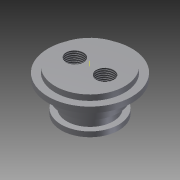
# Autodesk Inventor part: GL45 bottle cap insert with npt fittings
Saved by Autodesk Inventor 2011 (Build 150239000, 239)
## iProperties
Created: 2012-03-14
Part Number: GL45 bottle cap insert with npt fittings
Document SubType Name: Modeling
Designer: Marc
Density: 1 g/cm^3
Author: Marc
Autodesk Inventor part; units mm, degrees
ref_plane "YZ Plane" through (0, 0, 0) normal (1, 0, 0) x (0, 1, 0)
ref_plane "XZ Plane" through (0, 0, 0) normal (0, 1, 0) x (-1, 0, 0)
ref_plane "XY Plane" through (0, 0, 0) normal (0, 0, 1) x (1, 0, 0)
sketch "Sketch1" plane through (0, 0, 0) normal (0, 0, 1) x (1, 0, 0)
  line L0 (0, 0) -> (-14.478, 0)
  line L1 (-14.478, 0) -> (-14.478, 2.54)
  line L2 (-14.478, 2.54) -> (-11.684, 2.54)
  line L3 (-11.684, 2.54) -> (-11.684, 7.62)
  line L4 (-11.684, 7.62) -> (-14.478, 7.62)
  line L5 (-14.478, 7.62) -> (-14.478, 15.24)
  line L6 (-14.478, 15.24) -> (-21.082, 15.24)
  line L7 (-21.082, 15.24) -> (-21.082, 18.034)
  line L8 (-21.082, 18.034) -> (-17.526, 18.034)
  line L9 (-17.526, 18.034) -> (-17.526, 20.828)
  line L10 (-17.526, 20.828) -> (0, 20.828)
  line L11 (0, 20.828) -> (0, 0)
  dimension "d0" = 17.526
  dimension "d1" = 21.082
  dimension "d2" = 14.478
  dimension "d3" = 11.684
  dimension "d4" = 2.794
  dimension "d5" = 5.588
  dimension "d7" = 18.288
  dimension "d8" = 13.208
  dimension "d9" = 20.828
  constraints: 24 end point, 9 parallel, 2 collinear, 1 horizontal, 1 perpendicular
  measures "d0" distance of L9.end L10.end
  measures "d1" distance between parallel lines of L11 L7
  measures "d2" distance between parallel lines of L5 L11
  measures "d3" distance between parallel lines of L11 L3
  measures "d4" distance of L8.end L9.end
  measures "d5" distance between parallel lines of L6 L10
  measures "d7" distance between parallel lines of L2 L10
  measures "d8" distance between parallel lines of L10 L4
  measures "d9" distance between parallel lines of L0 L10
revolve "Revolution1" add sketch "Sketch1" angle 360 about axis through (0, 20.828, 0) along (0, -1, 0)
sketch "Sketch2" plane through (0, 20.828, 0) normal (0, 1, 0) x (1, 0, 0)
  circle A0 centre (0, 0) radius 14.478 projected
  circle A1 centre (0, 0) radius 11.684 projected
  line L0 (-29.5148, 0) -> (29.5148, 0) projected
  line L1 (14.0358, 0) -> (10.8279, -5.5563) construction
  line L2 (10.8279, -5.5563) -> (4.4121, -5.5563) construction
  line L3 (4.4121, -5.5563) -> (1.2042, 0) construction
  line L4 (1.2042, 0) -> (4.4121, 5.5562) construction
  line L5 (4.4121, 5.5562) -> (10.8279, 5.5563) construction
  line L6 (10.8279, 5.5563) -> (14.0358, 0) construction
  circle A2 centre (7.62, 0) radius 5.1435 construction
  circle A3 centre (7.62, 0) radius 3.175 construction
  line L7 (0, 0) -> (0, 8.1395) construction
  circle A4 centre (-7.62, 0) radius 5.1435 construction
  circle A5 centre (-7.62, 0) radius 3.175 construction
  line L8 (-0.2877, 0) -> (-3.9538, -6.35) construction
  line L9 (-3.9538, -6.35) -> (-11.2862, -6.35) construction
  line L10 (-11.2862, -6.35) -> (-14.9523, 0) construction
  line L11 (-14.9523, 0) -> (-11.2862, 6.35) construction
  line L12 (-11.2862, 6.35) -> (-3.9538, 6.35) construction
  line L13 (-3.9538, 6.35) -> (-0.2877, 0) construction
  dimension "d11" = 11.1125
  dimension "d12" = 10.287
  dimension "d13" = 6.35
  dimension "d15" = 12.7
  dimension "d17" = 15.24
  constraints: 26 end point, 7 coincident, 4 centre point, 3 point on line, 3 symmetric about line, 1 perpendicular, 28 other
  measures "d11" distance between parallel lines of L2 L5
  measures "d12" diameter of A2
  measures "d13" diameter of A3
  measures "d15" distance between parallel lines of L9 L12
  measures "d17" distance of point (7.62, 0) A5.centre
hole "Hole1" at (7.62, 20.828, 0) at (-7.62, 20.828, 0) direction (0, -1, 0) diameter 6.5278 end through all
sketch "Sketch3" plane through (0, 20.828, 0) normal (0, 1, 0) x (1, 0, 0)
  circle A0 centre (-7.62, 0) radius 3.2639 projected
  circle A1 centre (7.62, 0) radius 3.2639 projected
  constraints: 2 coincident
hole "Hole2" at (-7.62, 20.828, 0) at (7.62, 20.828, 0) direction (0, -1, 0) diameter 7.9502 depth 9.525 tip angle 118 taper from width 8.739 to width 8.3058 over 6.9342 thread size "1/8" designation "1/8 - 27 NPT" standard "NPT"
body "Solid1"
